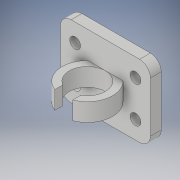
# Autodesk Inventor part: uchwyt_przewody
Saved by Autodesk Inventor 2019 (Build 230136000, 136)
## iProperties
Created: 2018-10-26
Part Number: uchwyt_przewody
Material: Ogólny
Document SubType Name: Modeling
Designer: user
Density: 1 g/cm^3
Appearance: Domyślna
Author: user
Autodesk Inventor part; units mm, degrees
ref_plane "YZ Plane" through (0, 0, 0) normal (1, 0, 0) x (0, 1, 0)
ref_plane "XZ Plane" through (0, 0, 0) normal (0, 1, 0) x (-1, 0, 0)
ref_plane "XY Plane" through (0, 0, 0) normal (0, 0, 1) x (1, 0, 0)
sketch "Szkic1" plane through (0, 0, 0) normal (0, 0, 1) x (1, 0, 0)
  line L0 (-12.5, -10) -> (12.5, -10)
  line L1 (12.5, -10) -> (12.5, 10)
  line L2 (12.5, 10) -> (-12.5, 10)
  line L3 (-12.5, 10) -> (-12.5, -10)
  line L4 (-12.5, -10) -> (12.5, 10) construction
  line L5 (12.5, -10) -> (-12.5, 10) construction
  point P0 (0, 0)
  dimension "d0" = 25
  dimension "d1" = 20
  constraints: 12 end point, 2 midpoint, 2 parallel, 1 horizontal, 1 perpendicular
  measures "d0" distance of L2.end L1.end
  measures "d1" distance of L1.end L0.end
extrude "Wyciągnięcie proste1" add sketch "Szkic1" along normal blind 3
sketch "Szkic2" plane through (0, 0, 0) normal (0, 1, 0) x (-1, 0, 0)
  circle A0 centre (0, 8) radius 7
  line L0 (12.5, 3) -> (-12.5, 3) projected
  line L1 (12.5, 0) -> (-12.5, 0) projected
  circle A1 centre (0, 8) radius 5
  line L2 (4.899, 3) -> (-4.899, 3)
  point P0 (0, 0)
  point P1 (0, 0)
  dimension "d4" = 14
  dimension "d5" = 10
  constraints: 2 centre point, 2 end point, 2 point on circle, 2 point on line, 1 coincident, 1 midpoint, 1 tangent, 1 vertical alignment
  measures "d4" diameter of A0
  measures "d5" diameter of A1
extrude "Wyciągnięcie proste2" add sketch "Szkic2" along normal mid plane 5 contours A0 L0 picked at (6.263, 8.5684)
sketch "Szkic3" plane through (-12.5, 10, 0) normal (0, 1, 0) x (1, 0, 0)
  line L0 (10, -16) -> (15, -16)
  line L1 (15, -16) -> (15, -12)
  line L2 (15, -12) -> (10, -12)
  line L3 (10, -12) -> (10, -16)
  line L4 (10, -16) -> (15, -12) construction
  line L5 (15, -16) -> (10, -12) construction
  circle A0 centre (12.5, -8) radius 5 projected
  line L6 (25, 0) -> (0, 0) projected
  point P0 (12.5, 0)
  point P1 (12.5, -14)
  point P2 (12.5, -14)
  point P3 (12.5, 0)
  dimension "d8" = 5
  dimension "d9" = 4
  dimension "d10" = 6
  constraints: 12 end point, 4 midpoint, 2 parallel, 1 horizontal, 1 perpendicular, 1 vertical alignment
  measures "d8" distance of L2.end L1.end
  measures "d9" distance of L1.end L0.end
  measures "d10" distance of A0.centre point (12.5, -14)
extrude "Wyciągnięcie proste3" cut sketch "Szkic3" against normal blind 20 contours L3 A0 L1 L0 | L3 L2 L1 A0 picked at (12.3258, -12.3242)
sketch "Szkic5" plane through (0, 0, 0) normal (0, 0, -1) x (-1, 0, 0)
  line L0 (12.5, 10) -> (12.5, -10) projected
  line L1 (-12.5, 10) -> (12.5, 10) projected
  line L2 (-12.5, -10) -> (-12.5, 10) projected
  line L3 (-12.5, 0) -> (12.5, 0) construction
  line L4 (0, 10) -> (0, -10) construction
  line L5 (12.5, -10) -> (-12.5, -10) projected
  point P0 (0, 0)
  point P1 (8.375, 5)
  point P2 (8.375, -5)
  point P3 (-8.375, 5)
  point P4 (-8.375, -5)
  dimension "d22" = 4.125
  dimension "d23" = 5
  constraints: 4 end point, 4 midpoint, 3 symmetric about line
  measures "d22" distance from line of L0 point (8.375, 5)
  measures "d23" distance from line of L1 point (8.375, 5)
hole "Otwór2" at (-8.375, 5, 0) at (-8.375, -5, 0) at (8.375, 5, 0) at (8.375, -5, 0) direction (0, 0, 1) diameter 3 end through all
fillet "Zaokrąglenie1" radius 3 4 edges at (-12.5, -10, 1.5) (-12.5, 10, 1.5) (12.5, 10, 1.5) (12.5, -10, 1.5)
